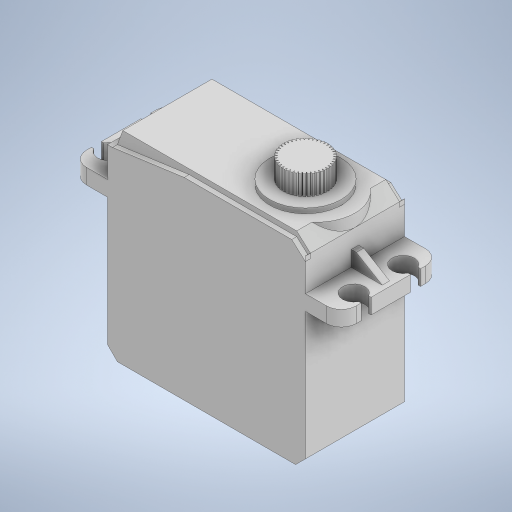
# Autodesk Inventor part: сервопривод DS3240
Saved by Autodesk Inventor 2023.2 (Build 272271000, 271)
## iProperties
Created: 2024-07-29
Part Number: сервопривод DS3240
Material: Типовые
Document SubType Name: Modeling
Designer: End_Ways
Density: 1 g/cm^3
Appearance: По умолчанию
Author: End_Ways
Autodesk Inventor part; units mm, degrees
ref_plane "YZ Plane" through (0, 0, 0) normal (1, 0, 0) x (0, 1, 0)
ref_plane "XZ Plane" through (0, 0, 0) normal (0, 1, 0) x (-1, 0, 0)
ref_plane "XY Plane" through (0, 0, 0) normal (0, 0, 1) x (1, 0, 0)
sketch "Эскиз1" plane through (0, 0, 0) normal (0, 0, 1) x (1, 0, 0)
  line L0 (0, 0) -> (20, 0)
  line L1 (20, 0) -> (20, 40)
  line L2 (20, 40) -> (0, 40)
  line L3 (0, 40) -> (0, 0)
  dimension "d0" = 20
  dimension "d1" = 40
  constraints: 8 end point, 2 parallel, 1 horizontal, 1 perpendicular
  measures "d0" distance of L2.end L1.end
  measures "d1" distance of L1.end L0.end
extrude "Выдавливание1" add sketch "Эскиз1" along normal blind 20
sketch "Эскиз2" plane through (0, 0, 20) normal (0, 0, 1) x (1, 0, 0)
  line L0 (0, 40) -> (0, 0) construction
  line L1 (0, 0) -> (0, 27.8) construction
  line L2 (0, 27.8) -> (-7.25, 27.8)
  line L3 (-7.25, 27.8) -> (-7.25, 30.9)
  line L4 (-7.25, 30.9) -> (0, 30.9)
  line L5 (0, 30.9) -> (0, 27.8)
  line L6 (20, 0) -> (20, 40) projected
  line L7 (20, 30.9) -> (20, 27.8)
  dimension "d4" = 27.8
  dimension "d5" = 7.25
  dimension "d6" = 3.1
  constraints: 12 end point, 2 parallel, 2 point on line, 1 horizontal, 1 perpendicular
  measures "d4" distance of L0.end L1.end
  measures "d5" distance of L3.end L4.end
  measures "d6" distance of L2.end L3.end
extrude "Выдавливание2" add sketch "Эскиз2" against normal blind 20
sketch "Эскиз3" plane through (-7.25, 30.9, 20) normal (0, 1, 0) x (1, 0, 0)
  circle A0 centre (2.5, 5) radius 2.25 construction
  circle A1 centre (2.5, 15) radius 2.25 construction
  line L0 (0, 20) -> (7.25, 20) construction
  line L1 (7.25, 20) -> (7.25, 0) construction
  circle A2 centre (2.5, 15) radius 2.25
  circle A3 centre (2.5, 5) radius 2.25
  line L2 (0, 0) -> (0, 20) construction
  line L3 (0, 16) -> (0.4844, 16) construction
  line L4 (0.4844, 16) -> (0.4844, 14) construction
  line L5 (0.4844, 14) -> (0, 14) construction
  line L6 (0, 14) -> (0, 16) construction
  line L7 (0, 16) -> (0.4844, 16)
  line L8 (0.4844, 16) -> (0.4844, 14)
  line L9 (0.4844, 14) -> (0, 14)
  line L10 (0, 14) -> (0, 16)
  line L11 (0, 6) -> (0.4844, 6)
  line L12 (0.4844, 6) -> (0.4844, 4)
  line L13 (0.4844, 4) -> (0, 4)
  line L14 (0, 4) -> (0, 6)
  point P0 (2.5, 17.25)
  point P1 (0.4844, 16)
  point P2 (0.4844, 6)
  dimension "d10" = 4.5
  dimension "d11" = 4.5
  dimension "d12" = 10
  dimension "d13" = 5
  dimension "d14" = 4.75
  dimension "d15" = 4.75
  dimension "d16" = 4
  dimension "d18" = 1
  constraints: 24 end point, 6 parallel, 3 centre point, 3 horizontal, 3 perpendicular, 2 coincident, 2 point on circle, 2 point on line, 1 concentric, 4 other
  measures "d10" diameter of A0
  measures "d11" diameter of A1
  measures "d12" distance of A0.centre A1.centre
  measures "d13" distance from line of L0 A1.centre
  measures "d14" distance from line of L1 A1.centre
  measures "d15" distance from line of L1 A0.centre
  measures "d16" distance of L3.start L0.start
  measures "d18" vertical distance of L11.end A0.centre
extrude "Выдавливание3" cut sketch "Эскиз3" against normal blind 20
mirror "Зеркальное отражение1" about plane through (20, 0, 0) normal (1, 0, 0) of "Выдавливание2", "Выдавливание1", "Выдавливание3"
fillet "Сопряжение1" radius 3 4 edges at (-7.25, 29.35, 20) (-7.25, 29.35, 0) (47.25, 29.35, 20) (47.25, 29.35, 0)
chamfer "Фаска1" distance 2 angle 45 2 edges at (40, 0, 10) (0, 0, 10)
sketch "Эскиз4" plane through (0, 40, 20) normal (0, 1, 0) x (1, 0, 0)
  line L0 (40, 20) -> (40, 0) construction
  line L1 (0, 0) -> (40, 0) construction
  line L2 (47.25, 6) -> (47.25, 14) construction
  line L3 (-7.25, 6) -> (-6.7656, 6) construction
  line L4 (47.25, 6) -> (-7.25, 6) construction
  circle A0 centre (30, 10) radius 4
  line L5 (30, 14.4415) -> (29.8, 14.4415)
  line L6 (29.8, 14.4415) -> (29.7204, 13.9902)
  line L7 (30, 14.4415) -> (30.2, 14.4415)
  line L8 (30.2, 14.4415) -> (30.2796, 13.9902)
  line L9 (29.5358, 14.4217) -> (29.6817, 13.9873)
  line L10 (29.338, 14.3919) -> (29.1403, 14.3621)
  line L11 (29.1403, 14.3621) -> (29.1288, 13.904)
  line L12 (29.338, 14.3919) -> (29.5358, 14.4217)
  line L13 (28.882, 14.3031) -> (29.091, 13.8953)
  line L14 (28.6908, 14.2442) -> (28.4997, 14.1852)
  line L15 (28.4997, 14.1852) -> (28.5567, 13.7305)
  line L16 (28.6908, 14.2442) -> (28.882, 14.3031)
  line L17 (28.2531, 14.0884) -> (28.5206, 13.7164)
  line L18 (28.0729, 14.0016) -> (27.8927, 13.9149)
  line L19 (27.8927, 13.9149) -> (28.0168, 13.4738)
  line L20 (28.0729, 14.0016) -> (28.2531, 14.0884)
  line L21 (27.6633, 13.7824) -> (27.9832, 13.4544)
  line L22 (27.498, 13.6697) -> (27.3328, 13.5571)
  line L23 (27.3328, 13.5571) -> (27.5212, 13.1394)
  line L24 (27.498, 13.6697) -> (27.6633, 13.7824)
  line L25 (27.1256, 13.3919) -> (27.4909, 13.1152)
  line L26 (26.979, 13.2558) -> (26.8324, 13.1198)
  line L27 (26.8324, 13.1198) -> (27.081, 12.7349)
  line L28 (26.979, 13.2558) -> (27.1256, 13.3919)
  line L29 (26.6522, 12.9256) -> (27.0546, 12.7064)
  line L30 (26.5275, 12.7692) -> (26.4028, 12.6129)
  line L31 (26.4028, 12.6129) -> (26.706, 12.2693)
  line L32 (26.5275, 12.7692) -> (26.6522, 12.9256)
  line L33 (26.2536, 12.3939) -> (26.6842, 12.2372)
  line L34 (26.1536, 12.2207) -> (26.0536, 12.0475)
  line L35 (26.0536, 12.0475) -> (26.4046, 11.753)
  line L36 (26.1536, 12.2207) -> (26.2536, 12.3939)
  line L37 (25.9386, 11.8088) -> (26.3877, 11.718)
  line L38 (25.8655, 11.6227) -> (25.7925, 11.4365)
  line L39 (25.7925, 11.4365) -> (26.1835, 11.1975)
  line L40 (25.8655, 11.6227) -> (25.9386, 11.8088)
  line L41 (25.7144, 11.1833) -> (26.172, 11.1605)
  line L42 (25.6699, 10.9883) -> (25.6254, 10.7933)
  line L43 (25.6254, 10.7933) -> (26.0476, 10.6153)
  line L44 (25.6699, 10.9883) -> (25.7144, 11.1833)
  line L45 (25.5859, 10.5314) -> (26.0418, 10.577)
  line L46 (25.5709, 10.3319) -> (25.556, 10.1325)
  line L47 (25.556, 10.1325) -> (26, 10.0194)
  line L48 (25.5709, 10.3319) -> (25.5859, 10.5314)
  line L49 (25.556, 9.8675) -> (26, 9.9806)
  line L50 (25.5709, 9.6681) -> (25.5859, 9.4686)
  line L51 (25.5859, 9.4686) -> (26.0418, 9.423)
  line L52 (25.5709, 9.6681) -> (25.556, 9.8675)
  line L53 (25.6254, 9.2067) -> (26.0476, 9.3847)
  line L54 (25.6699, 9.0117) -> (25.7144, 8.8167)
  line L55 (25.7144, 8.8167) -> (26.172, 8.8395)
  line L56 (25.6699, 9.0117) -> (25.6254, 9.2067)
  line L57 (25.7925, 8.5635) -> (26.1835, 8.8025)
  line L58 (25.8655, 8.3773) -> (25.9386, 8.1912)
  line L59 (25.9386, 8.1912) -> (26.3877, 8.282)
  line L60 (25.8655, 8.3773) -> (25.7925, 8.5635)
  line L61 (26.0536, 7.9525) -> (26.4046, 8.247)
  line L62 (26.1536, 7.7793) -> (26.2536, 7.6061)
  line L63 (26.2536, 7.6061) -> (26.6842, 7.7628)
  line L64 (26.1536, 7.7793) -> (26.0536, 7.9525)
  line L65 (26.4028, 7.3871) -> (26.706, 7.7307)
  line L66 (26.5275, 7.2308) -> (26.6522, 7.0744)
  line L67 (26.6522, 7.0744) -> (27.0546, 7.2936)
  line L68 (26.5275, 7.2308) -> (26.4028, 7.3871)
  line L69 (26.8324, 6.8802) -> (27.081, 7.2651)
  line L70 (26.979, 6.7442) -> (27.1256, 6.6081)
  line L71 (27.1256, 6.6081) -> (27.4909, 6.8848)
  line L72 (26.979, 6.7442) -> (26.8324, 6.8802)
  line L73 (27.3328, 6.4429) -> (27.5212, 6.8606)
  line L74 (27.498, 6.3303) -> (27.6633, 6.2176)
  line L75 (27.6633, 6.2176) -> (27.9832, 6.5456)
  line L76 (27.498, 6.3303) -> (27.3328, 6.4429)
  line L77 (27.8927, 6.0851) -> (28.0168, 6.5262)
  line L78 (28.0729, 5.9984) -> (28.2531, 5.9116)
  line L79 (28.2531, 5.9116) -> (28.5206, 6.2836)
  line L80 (28.0729, 5.9984) -> (27.8927, 6.0851)
  line L81 (28.4997, 5.8148) -> (28.5567, 6.2695)
  line L82 (28.6908, 5.7558) -> (28.882, 5.6969)
  line L83 (28.882, 5.6969) -> (29.091, 6.1047)
  line L84 (28.6908, 5.7558) -> (28.4997, 5.8148)
  line L85 (29.1403, 5.6379) -> (29.1288, 6.096)
  line L86 (29.338, 5.6081) -> (29.5358, 5.5783)
  line L87 (29.5358, 5.5783) -> (29.6817, 6.0127)
  line L88 (29.338, 5.6081) -> (29.1403, 5.6379)
  line L89 (29.8, 5.5585) -> (29.7204, 6.0098)
  line L90 (30, 5.5585) -> (30.2, 5.5585)
  line L91 (30.2, 5.5585) -> (30.2796, 6.0098)
  line L92 (30, 5.5585) -> (29.8, 5.5585)
  line L93 (30.4642, 5.5783) -> (30.3183, 6.0127)
  line L94 (30.662, 5.6081) -> (30.8597, 5.6379)
  line L95 (30.8597, 5.6379) -> (30.8712, 6.096)
  line L96 (30.662, 5.6081) -> (30.4642, 5.5783)
  line L97 (31.118, 5.6969) -> (30.909, 6.1047)
  line L98 (31.3092, 5.7558) -> (31.5003, 5.8148)
  line L99 (31.5003, 5.8148) -> (31.4433, 6.2695)
  line L100 (31.3092, 5.7558) -> (31.118, 5.6969)
  line L101 (31.7469, 5.9116) -> (31.4794, 6.2836)
  line L102 (31.9271, 5.9984) -> (32.1073, 6.0851)
  line L103 (32.1073, 6.0851) -> (31.9832, 6.5262)
  line L104 (31.9271, 5.9984) -> (31.7469, 5.9116)
  line L105 (32.3367, 6.2176) -> (32.0168, 6.5456)
  line L106 (32.502, 6.3303) -> (32.6672, 6.4429)
  line L107 (32.6672, 6.4429) -> (32.4788, 6.8606)
  line L108 (32.502, 6.3303) -> (32.3367, 6.2176)
  line L109 (32.8744, 6.6081) -> (32.5091, 6.8848)
  line L110 (33.021, 6.7442) -> (33.1676, 6.8802)
  line L111 (33.1676, 6.8802) -> (32.919, 7.2651)
  line L112 (33.021, 6.7442) -> (32.8744, 6.6081)
  line L113 (33.3478, 7.0744) -> (32.9454, 7.2936)
  line L114 (33.4725, 7.2308) -> (33.5972, 7.3871)
  line L115 (33.5972, 7.3871) -> (33.294, 7.7307)
  line L116 (33.4725, 7.2308) -> (33.3478, 7.0744)
  line L117 (33.7464, 7.6061) -> (33.3158, 7.7628)
  line L118 (33.8464, 7.7793) -> (33.9464, 7.9525)
  line L119 (33.9464, 7.9525) -> (33.5954, 8.247)
  line L120 (33.8464, 7.7793) -> (33.7464, 7.6061)
  line L121 (34.0614, 8.1912) -> (33.6123, 8.282)
  line L122 (34.1345, 8.3773) -> (34.2075, 8.5635)
  line L123 (34.2075, 8.5635) -> (33.8165, 8.8025)
  line L124 (34.1345, 8.3773) -> (34.0614, 8.1912)
  line L125 (34.2856, 8.8167) -> (33.828, 8.8395)
  line L126 (34.3301, 9.0117) -> (34.3746, 9.2067)
  line L127 (34.3746, 9.2067) -> (33.9524, 9.3847)
  line L128 (34.3301, 9.0117) -> (34.2856, 8.8167)
  line L129 (34.4141, 9.4686) -> (33.9582, 9.423)
  line L130 (34.4291, 9.6681) -> (34.444, 9.8675)
  line L131 (34.444, 9.8675) -> (34, 9.9806)
  line L132 (34.4291, 9.6681) -> (34.4141, 9.4686)
  line L133 (34.444, 10.1325) -> (34, 10.0194)
  line L134 (34.4291, 10.3319) -> (34.4141, 10.5314)
  line L135 (34.4141, 10.5314) -> (33.9582, 10.577)
  line L136 (34.4291, 10.3319) -> (34.444, 10.1325)
  line L137 (34.3746, 10.7933) -> (33.9524, 10.6153)
  line L138 (34.3301, 10.9883) -> (34.2856, 11.1833)
  line L139 (34.2856, 11.1833) -> (33.828, 11.1605)
  line L140 (34.3301, 10.9883) -> (34.3746, 10.7933)
  line L141 (34.2075, 11.4365) -> (33.8165, 11.1975)
  line L142 (34.1345, 11.6227) -> (34.0614, 11.8088)
  line L143 (34.0614, 11.8088) -> (33.6123, 11.718)
  line L144 (34.1345, 11.6227) -> (34.2075, 11.4365)
  line L145 (33.9464, 12.0475) -> (33.5954, 11.753)
  line L146 (33.8464, 12.2207) -> (33.7464, 12.3939)
  line L147 (33.7464, 12.3939) -> (33.3158, 12.2372)
  line L148 (33.8464, 12.2207) -> (33.9464, 12.0475)
  line L149 (33.5972, 12.6129) -> (33.294, 12.2693)
  line L150 (33.4725, 12.7692) -> (33.3478, 12.9256)
  line L151 (33.3478, 12.9256) -> (32.9454, 12.7064)
  line L152 (33.4725, 12.7692) -> (33.5972, 12.6129)
  line L153 (33.1676, 13.1198) -> (32.919, 12.7349)
  line L154 (33.021, 13.2558) -> (32.8744, 13.3919)
  line L155 (32.8744, 13.3919) -> (32.5091, 13.1152)
  line L156 (33.021, 13.2558) -> (33.1676, 13.1198)
  line L157 (32.6672, 13.5571) -> (32.4788, 13.1394)
  line L158 (32.502, 13.6697) -> (32.3367, 13.7824)
  line L159 (32.3367, 13.7824) -> (32.0168, 13.4544)
  line L160 (32.502, 13.6697) -> (32.6672, 13.5571)
  line L161 (32.1073, 13.9149) -> (31.9832, 13.4738)
  line L162 (31.9271, 14.0016) -> (31.7469, 14.0884)
  line L163 (31.7469, 14.0884) -> (31.4794, 13.7164)
  line L164 (31.9271, 14.0016) -> (32.1073, 13.9149)
  line L165 (31.5003, 14.1852) -> (31.4433, 13.7305)
  line L166 (31.3092, 14.2442) -> (31.118, 14.3031)
  line L167 (31.118, 14.3031) -> (30.909, 13.8953)
  line L168 (31.3092, 14.2442) -> (31.5003, 14.1852)
  line L169 (30.8597, 14.3621) -> (30.8712, 13.904)
  line L170 (30.662, 14.3919) -> (30.4642, 14.4217)
  line L171 (30.4642, 14.4217) -> (30.3183, 13.9873)
  line L172 (30.662, 14.3919) -> (30.8597, 14.3621)
  point P0 (0, 20)
  point P1 (29.6817, 6.0127)
  point P2 (29.1288, 6.096)
  point P3 (27.9832, 6.5456)
  point P4 (27.5212, 6.8606)
  point P5 (29.091, 6.1047)
  point P6 (28.5567, 6.2695)
  dimension "d25" = 10
  dimension "d26" = 10
  dimension "d50" = 0.2
  dimension "d51" = 100
  dimension "d52" = 0.2
  dimension "d55" = 360
  constraints: 338 end point, 4 horizontal, 1 coincident, 382 other
  measures "d25" distance from line of L0 point (30, 10)
  measures "d26" distance from line of L1 point (30, 10)
  measures "d50" distance of L5.start L5.end
  measures "d51" angle of L6 L5
  measures "d52" distance of L5.start L7.end
extrude "Выдавливание4" add sketch "Эскиз4" along normal blind 5
sketch "Эскиз5" plane through (0, 40, 20) normal (0, 1, 0) x (1, 0, 0)
  line L0 (47.25, 4) -> (25.9505, 4) construction
  arc A0 (33.5954, 8.247) -> (33.6123, 8.282) centre (30, 10) ccw projected
  circle A1 centre (30, 10) radius 7.2387
  line L1 (33.6123, 8.282) -> (34.0614, 8.1912) projected
  line L2 (34.0614, 8.1912) -> (34.2075, 8.5635) projected
  line L3 (34.2075, 8.5635) -> (33.8165, 8.8025) projected
  arc A2 (33.8165, 8.8025) -> (33.828, 8.8395) centre (30, 10) ccw projected
  line L4 (33.828, 8.8395) -> (34.2856, 8.8167) projected
  line L5 (34.2856, 8.8167) -> (34.3746, 9.2067) projected
  line L6 (34.3746, 9.2067) -> (33.9524, 9.3847) projected
  arc A3 (33.9524, 9.3847) -> (33.9582, 9.423) centre (30, 10) ccw projected
  line L7 (33.9582, 9.423) -> (34.4141, 9.4686) projected
  line L8 (34.4141, 9.4686) -> (34.444, 9.8675) projected
  line L9 (34.444, 9.8675) -> (34, 9.9806) projected
  arc A4 (34, 9.9806) -> (34, 10.0194) centre (30, 10) ccw projected
  line L10 (34, 10.0194) -> (34.444, 10.1325) projected
  line L11 (34.444, 10.1325) -> (34.4141, 10.5314) projected
  line L12 (34.4141, 10.5314) -> (33.9582, 10.577) projected
  arc A5 (33.9582, 10.577) -> (33.9524, 10.6153) centre (30, 10) ccw projected
  line L13 (33.9524, 10.6153) -> (34.3746, 10.7933) projected
  line L14 (34.3746, 10.7933) -> (34.2856, 11.1833) projected
  line L15 (34.2856, 11.1833) -> (33.828, 11.1605) projected
  arc A6 (33.828, 11.1605) -> (33.8165, 11.1975) centre (30, 10) ccw projected
  line L16 (33.8165, 11.1975) -> (34.2075, 11.4365) projected
  line L17 (34.2075, 11.4365) -> (34.0614, 11.8088) projected
  line L18 (34.0614, 11.8088) -> (33.6123, 11.718) projected
  arc A7 (33.6123, 11.718) -> (33.5954, 11.753) centre (30, 10) ccw projected
  line L19 (33.5954, 11.753) -> (33.9464, 12.0475) projected
  line L20 (33.9464, 12.0475) -> (33.7464, 12.3939) projected
  line L21 (33.7464, 12.3939) -> (33.3158, 12.2372) projected
  arc A8 (33.3158, 12.2372) -> (33.294, 12.2693) centre (30, 10) ccw projected
  line L22 (33.294, 12.2693) -> (33.5972, 12.6129) projected
  line L23 (33.5972, 12.6129) -> (33.3478, 12.9256) projected
  line L24 (33.3478, 12.9256) -> (32.9454, 12.7064) projected
  arc A9 (32.9454, 12.7064) -> (32.919, 12.7349) centre (30, 10) ccw projected
  line L25 (32.919, 12.7349) -> (33.1676, 13.1198) projected
  line L26 (33.1676, 13.1198) -> (32.8744, 13.3919) projected
  line L27 (32.8744, 13.3919) -> (32.5091, 13.1152) projected
  arc A10 (32.5091, 13.1152) -> (32.4788, 13.1394) centre (30, 10) ccw projected
  line L28 (32.4788, 13.1394) -> (32.6672, 13.5571) projected
  line L29 (32.6672, 13.5571) -> (32.3367, 13.7824) projected
  line L30 (32.3367, 13.7824) -> (32.0168, 13.4544) projected
  arc A11 (32.0168, 13.4544) -> (31.9832, 13.4738) centre (30, 10) ccw projected
  line L31 (31.9832, 13.4738) -> (32.1073, 13.9149) projected
  line L32 (32.1073, 13.9149) -> (31.7469, 14.0884) projected
  line L33 (31.7469, 14.0884) -> (31.4794, 13.7164) projected
  arc A12 (31.4794, 13.7164) -> (31.4433, 13.7305) centre (30, 10) ccw projected
  line L34 (31.4433, 13.7305) -> (31.5003, 14.1852) projected
  line L35 (31.5003, 14.1852) -> (31.118, 14.3031) projected
  line L36 (31.118, 14.3031) -> (30.909, 13.8953) projected
  arc A13 (30.909, 13.8953) -> (30.8712, 13.904) centre (30, 10) ccw projected
  line L37 (30.8712, 13.904) -> (30.8597, 14.3621) projected
  line L38 (30.8597, 14.3621) -> (30.4642, 14.4217) projected
  line L39 (30.4642, 14.4217) -> (30.3183, 13.9873) projected
  arc A14 (30.3183, 13.9873) -> (30.2796, 13.9902) centre (30, 10) ccw projected
  line L40 (30.2796, 13.9902) -> (30.2, 14.4415) projected
  line L41 (30.2, 14.4415) -> (29.8, 14.4415) projected
  line L42 (29.8, 14.4415) -> (29.7204, 13.9902) projected
  arc A15 (29.7204, 13.9902) -> (29.6817, 13.9873) centre (30, 10) ccw projected
  line L43 (29.6817, 13.9873) -> (29.5358, 14.4217) projected
  line L44 (29.5358, 14.4217) -> (29.1403, 14.3621) projected
  line L45 (29.1403, 14.3621) -> (29.1288, 13.904) projected
  arc A16 (29.1288, 13.904) -> (29.091, 13.8953) centre (30, 10) ccw projected
  line L46 (29.091, 13.8953) -> (28.882, 14.3031) projected
  line L47 (28.882, 14.3031) -> (28.4997, 14.1852) projected
  line L48 (28.4997, 14.1852) -> (28.5567, 13.7305) projected
  arc A17 (28.5567, 13.7305) -> (28.5206, 13.7164) centre (30, 10) ccw projected
  line L49 (28.5206, 13.7164) -> (28.2531, 14.0884) projected
  line L50 (28.2531, 14.0884) -> (27.8927, 13.9149) projected
  line L51 (27.8927, 13.9149) -> (28.0168, 13.4738) projected
  arc A18 (28.0168, 13.4738) -> (27.9832, 13.4544) centre (30, 10) ccw projected
  line L52 (27.9832, 13.4544) -> (27.6633, 13.7824) projected
  line L53 (27.6633, 13.7824) -> (27.3328, 13.5571) projected
  line L54 (27.3328, 13.5571) -> (27.5212, 13.1394) projected
  arc A19 (27.5212, 13.1394) -> (27.4909, 13.1152) centre (30, 10) ccw projected
  line L55 (27.4909, 13.1152) -> (27.1256, 13.3919) projected
  line L56 (27.1256, 13.3919) -> (26.8324, 13.1198) projected
  line L57 (26.8324, 13.1198) -> (27.081, 12.7349) projected
  arc A20 (27.081, 12.7349) -> (27.0546, 12.7064) centre (30, 10) ccw projected
  line L58 (27.0546, 12.7064) -> (26.6522, 12.9256) projected
  line L59 (26.6522, 12.9256) -> (26.4028, 12.6129) projected
  line L60 (26.4028, 12.6129) -> (26.706, 12.2693) projected
  arc A21 (26.706, 12.2693) -> (26.6842, 12.2372) centre (30, 10) ccw projected
  line L61 (26.6842, 12.2372) -> (26.2536, 12.3939) projected
  line L62 (26.2536, 12.3939) -> (26.0536, 12.0475) projected
  line L63 (26.0536, 12.0475) -> (26.4046, 11.753) projected
  arc A22 (26.4046, 11.753) -> (26.3877, 11.718) centre (30, 10) ccw projected
  line L64 (26.3877, 11.718) -> (25.9386, 11.8088) projected
  line L65 (25.9386, 11.8088) -> (25.7925, 11.4365) projected
  line L66 (25.7925, 11.4365) -> (26.1835, 11.1975) projected
  arc A23 (26.1835, 11.1975) -> (26.172, 11.1605) centre (30, 10) ccw projected
  line L67 (26.172, 11.1605) -> (25.7144, 11.1833) projected
  line L68 (25.7144, 11.1833) -> (25.6254, 10.7933) projected
  line L69 (25.6254, 10.7933) -> (26.0476, 10.6153) projected
  arc A24 (26.0476, 10.6153) -> (26.0418, 10.577) centre (30, 10) ccw projected
  line L70 (26.0418, 10.577) -> (25.5859, 10.5314) projected
  line L71 (25.5859, 10.5314) -> (25.556, 10.1325) projected
  line L72 (25.556, 10.1325) -> (26, 10.0194) projected
  arc A25 (26, 10.0194) -> (26, 9.9806) centre (30, 10) ccw projected
  line L73 (26, 9.9806) -> (25.556, 9.8675) projected
  line L74 (25.556, 9.8675) -> (25.5859, 9.4686) projected
  line L75 (25.5859, 9.4686) -> (26.0418, 9.423) projected
  arc A26 (26.0418, 9.423) -> (26.0476, 9.3847) centre (30, 10) ccw projected
  line L76 (26.0476, 9.3847) -> (25.6254, 9.2067) projected
  line L77 (25.6254, 9.2067) -> (25.7144, 8.8167) projected
  line L78 (25.7144, 8.8167) -> (26.172, 8.8395) projected
  arc A27 (26.172, 8.8395) -> (26.1835, 8.8025) centre (30, 10) ccw projected
  line L79 (26.1835, 8.8025) -> (25.7925, 8.5635) projected
  line L80 (25.7925, 8.5635) -> (25.9386, 8.1912) projected
  line L81 (25.9386, 8.1912) -> (26.3877, 8.282) projected
  arc A28 (26.3877, 8.282) -> (26.4046, 8.247) centre (30, 10) ccw projected
  line L82 (26.4046, 8.247) -> (26.0536, 7.9525) projected
  line L83 (26.0536, 7.9525) -> (26.2536, 7.6061) projected
  line L84 (26.2536, 7.6061) -> (26.6842, 7.7628) projected
  arc A29 (26.6842, 7.7628) -> (26.706, 7.7307) centre (30, 10) ccw projected
  line L85 (26.706, 7.7307) -> (26.4028, 7.3871) projected
  line L86 (26.4028, 7.3871) -> (26.6522, 7.0744) projected
  line L87 (26.6522, 7.0744) -> (27.0546, 7.2936) projected
  arc A30 (27.0546, 7.2936) -> (27.081, 7.2651) centre (30, 10) ccw projected
  line L88 (27.081, 7.2651) -> (26.8324, 6.8802) projected
  line L89 (26.8324, 6.8802) -> (27.1256, 6.6081) projected
  line L90 (27.1256, 6.6081) -> (27.4909, 6.8848) projected
  arc A31 (27.4909, 6.8848) -> (27.5212, 6.8606) centre (30, 10) ccw projected
  line L91 (27.5212, 6.8606) -> (27.3328, 6.4429) projected
  line L92 (27.3328, 6.4429) -> (27.6633, 6.2176) projected
  line L93 (27.6633, 6.2176) -> (27.9832, 6.5456) projected
  arc A32 (27.9832, 6.5456) -> (28.0168, 6.5262) centre (30, 10) ccw projected
  line L94 (28.0168, 6.5262) -> (27.8927, 6.0851) projected
  line L95 (27.8927, 6.0851) -> (28.2531, 5.9116) projected
  line L96 (28.2531, 5.9116) -> (28.5206, 6.2836) projected
  arc A33 (28.5206, 6.2836) -> (28.5567, 6.2695) centre (30, 10) ccw projected
  line L97 (28.5567, 6.2695) -> (28.4997, 5.8148) projected
  line L98 (28.4997, 5.8148) -> (28.882, 5.6969) projected
  line L99 (28.882, 5.6969) -> (29.091, 6.1047) projected
  arc A34 (29.091, 6.1047) -> (29.1288, 6.096) centre (30, 10) ccw projected
  line L100 (29.1288, 6.096) -> (29.1403, 5.6379) projected
  line L101 (29.1403, 5.6379) -> (29.5358, 5.5783) projected
  line L102 (29.5358, 5.5783) -> (29.6817, 6.0127) projected
  arc A35 (29.6817, 6.0127) -> (29.7204, 6.0098) centre (30, 10) ccw projected
  line L103 (29.7204, 6.0098) -> (29.8, 5.5585) projected
  line L104 (29.8, 5.5585) -> (30.2, 5.5585) projected
  line L105 (30.2, 5.5585) -> (30.2796, 6.0098) projected
  arc A36 (30.2796, 6.0098) -> (30.3183, 6.0127) centre (30, 10) ccw projected
  line L106 (30.3183, 6.0127) -> (30.4642, 5.5783) projected
  line L107 (30.4642, 5.5783) -> (30.8597, 5.6379) projected
  line L108 (30.8597, 5.6379) -> (30.8712, 6.096) projected
  arc A37 (30.8712, 6.096) -> (30.909, 6.1047) centre (30, 10) ccw projected
  line L109 (30.909, 6.1047) -> (31.118, 5.6969) projected
  line L110 (31.118, 5.6969) -> (31.5003, 5.8148) projected
  line L111 (31.5003, 5.8148) -> (31.4433, 6.2695) projected
  arc A38 (31.4433, 6.2695) -> (31.4794, 6.2836) centre (30, 10) ccw projected
  line L112 (31.4794, 6.2836) -> (31.7469, 5.9116) projected
  line L113 (31.7469, 5.9116) -> (32.1073, 6.0851) projected
  line L114 (32.1073, 6.0851) -> (31.9832, 6.5262) projected
  arc A39 (31.9832, 6.5262) -> (32.0168, 6.5456) centre (30, 10) ccw projected
  line L115 (32.0168, 6.5456) -> (32.3367, 6.2176) projected
  line L116 (32.3367, 6.2176) -> (32.6672, 6.4429) projected
  line L117 (32.6672, 6.4429) -> (32.4788, 6.8606) projected
  arc A40 (32.4788, 6.8606) -> (32.5091, 6.8848) centre (30, 10) ccw projected
  line L118 (32.5091, 6.8848) -> (32.8744, 6.6081) projected
  line L119 (32.8744, 6.6081) -> (33.1676, 6.8802) projected
  line L120 (33.1676, 6.8802) -> (32.919, 7.2651) projected
  arc A41 (32.919, 7.2651) -> (32.9454, 7.2936) centre (30, 10) ccw projected
  line L121 (32.9454, 7.2936) -> (33.3478, 7.0744) projected
  line L122 (33.3478, 7.0744) -> (33.5972, 7.3871) projected
  line L123 (33.5972, 7.3871) -> (33.294, 7.7307) projected
  arc A42 (33.294, 7.7307) -> (33.3158, 7.7628) centre (30, 10) ccw projected
  line L124 (33.3158, 7.7628) -> (33.7464, 7.6061) projected
  line L125 (33.7464, 7.6061) -> (33.9464, 7.9525) projected
  line L126 (33.9464, 7.9525) -> (33.5954, 8.247) projected
  point P0 (0, 20)
  constraints: 2 end point, 1 coincident, 1 horizontal, 3 other
extrude "Выдавливание5" add sketch "Эскиз5" along normal blind 1 contours L126 L125 L124 A42 L123 L122 L121 A41 L120 L119 L118 A40 L117 L116 L115 A39 L114 L113 L112 A38 L111 L110 L109 A37 L108 L107 L106 A36 L105 L104 L103 A35 L102 L101 L100 A34 L99 L98 L97 A33 L96 L95 L94 A32 L93 L92 L91 A31 L90 L89 L88 A30 L87 L86 L85 A29 L84 L83 L82 A28 L81 L80 L79 A27 L78 L77 L76 A26 L75 L74 L73 A25 L72 L71 L70 A24 L69 L68 L67 A23 L66 L65 L64 A22 L63 L62 L61 A21 L60 L59 L58 A20 L57 L56 L55 A19 L54 L53 L52 A18 L51 L50 L49 A17 L48 L47 L46 A16 L45 L44 L43 A15 L42 L41 L40 A14 L39 L38 L37 A13 L36 L35 L34 A12 L33 L32 L31 A11 L30 L29 L28 A10 L27 L26 L25 A9 L24 L23 L22 A8 L21 L20 L19 A7 L18 L17 L16 A6 L15 L14 L13 A5 L12 L11 L10 A4 L9 L8 L7 A3 L6 L5 L4 A2 L3 L2 L1 A0 | A1
sketch "Эскиз6" plane through (0, 0, 20) normal (0, 0, 1) x (1, 0, 0)
  line L0 (0, 40) -> (40, 40) projected
  line L1 (37.2196, 40) -> (40, 37.4919)
  line L2 (40, 40) -> (40, 30.9) projected
  line L3 (0, 40) -> (1, 40) construction
  line L4 (1, 40) -> (1, 37) construction
  line L5 (1, 37) -> (0, 37) construction
  line L6 (0, 37) -> (0, 40) construction
  line L7 (1, 37) -> (2.0912, 40)
  line L8 (1, 37) -> (0, 37)
  line L9 (0, 40) -> (0, 30.9) projected
  line L10 (0, 40) -> (2.0912, 40)
  point P0 (0, 0)
  dimension "d35" = 1
  dimension "d36" = 3
  constraints: 16 end point, 3 point on line, 2 parallel, 2 perpendicular, 1 collinear, 1 horizontal
  measures "d35" distance of L4.end L5.end
  measures "d36" distance of L3.end L4.end
extrude "Выдавливание6" cut sketch "Эскиз6" against normal blind 30
sketch "Эскиз7" plane through (0, 40, 20) normal (0, 1, 0) x (1, 0, 0)
  circle A0 centre (30, 10) radius 7.2387 projected
  arc A1 (30, 2.7613) -> (30, 17.2387) centre (32.3801, 10) ccw
  line L0 (40, 20) -> (40, 0) projected
  point P0 (0, 20)
  constraints: 4 point on circle, 1 centre point, 1 tangent
extrude "Выдавливание7" add sketch "Эскиз7" against normal blind 4 contours A0 A1
sketch "Эскиз8" plane through (0, 0, 20) normal (0, 0, 1) x (1, 0, 0)
  line L0 (1, 37) -> (22.7518, 40)
  line L1 (2.0912, 40) -> (37.2196, 40) projected
  line L2 (1, 37) -> (2.0912, 40) projected
  line L3 (1, 37) -> (2.0912, 40)
  line L4 (22.7518, 40) -> (2.0912, 40)
  line L5 (23.6269, 39) -> (15.5012, 39)
  line L6 (23.6269, 39) -> (37.2196, 39)
  line L7 (37.2196, 39) -> (39.9796, 36.5103)
  line L8 (37.2196, 40) -> (40, 37.4919) projected
  line L9 (39.9796, 36.5103) -> (39.9796, 37.5103)
  point P0 (0, 0)
  dimension "d37" = 1
  constraints: 14 end point, 4 point on line, 2 collinear, 1 horizontal, 1 parallel, 1 perpendicular
  measures "d37" distance from line of L1 L5.start
extrude "Выдавливание8" cut sketch "Эскиз8" against normal blind 1
pattern_linear "Прямоуг.массив1" count 2 spacing 19 along (0, 0, -1) of "Выдавливание8"
ref_plane "РабПлоскость1" through (0, 0, 10) normal (0, 0, 1) x (1, 0, 0)
sketch "Эскиз9" plane through (0, 0, 10) normal (0, 0, 1) x (1, 0, 0)
  line L0 (44.25, 30.9) -> (47.25, 30.9) construction
  line L1 (40, 37.4919) -> (40, 30.9) construction
  line L2 (40, 34.0107) -> (41, 34.0107)
  line L3 (41, 34.0107) -> (46.25, 30.9)
  line L4 (46.25, 30.9) -> (40, 30.9)
  line L5 (40, 30.9) -> (40, 34.0107)
  line L6 (40, 34.0107) -> (0, 33.95) construction
  line L7 (0, 37) -> (0, 30.9) construction
  line L8 (0, 33.95) -> (-1, 33.9485)
  line L9 (-7.25, 30.9) -> (-6.25, 30.9) construction
  line L10 (-6.7656, 30.9) -> (-2.5, 30.9) construction
  line L11 (-6.25, 30.9) -> (-1, 33.9485)
  line L12 (-4.25, 30.9) -> (0, 30.9) projected
  line L13 (-6.25, 30.9) -> (0, 30.9)
  line L14 (0, 30.9) -> (0, 33.95)
  point P0 (0, 0)
  dimension "d44" = 1
  dimension "d45" = 1
  dimension "d46" = 1
  dimension "d47" = 1
  constraints: 20 end point, 4 point on line, 2 collinear, 2 horizontal, 1 coincident, 1 midpoint, 1 perpendicular
  measures "d44" distance of L3.end point (47.25, 30.9)
  measures "d45" distance of L2.start L2.end
  measures "d46" distance of L6.end L8.end
  measures "d47" distance of L9.start L9.end
extrude "Выдавливание9" add sketch "Эскиз9" along normal mid plane 1.5
